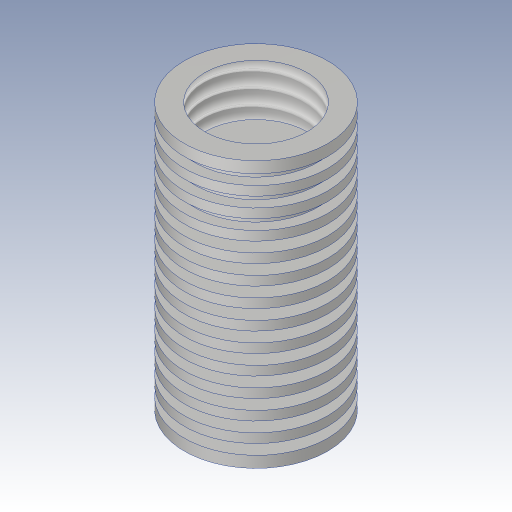
# Autodesk Inventor part: BT003_huenin20_23
Saved by Autodesk Inventor 2023.3 (Build 273359000, 359)
## iProperties
Company: HTBLA Kaindorf
RuleStatus: InUse
Created: 2023-08-12
Part Number: BT003_huenin20_23
Project: Fiberprinter-Hotend
Material: Aluminium 6061
Description: Coldend
Document SubType Name: Modeling
Designer: huenin20
Density: 2.7 g/cm^3
Appearance: Aluminium - flach
Mass: 5.305 g
Surface Area: 40.404 cm^2
Volume: 1.96481 cm^3
AfterDocNew0: iProperties-Editor_aufrufen
Author: nicob
Keywords: 2023
Autodesk Inventor part; units mm, degrees
ref_plane "YZ Plane" through (0, 0, 0) normal (1, 0, 0) x (0, 1, 0)
ref_plane "XZ Plane" through (0, 0, 0) normal (0, 1, 0) x (-1, 0, 0)
ref_plane "XY Plane" through (0, 0, 0) normal (0, 0, 1) x (1, 0, 0)
sketch "Skizze3" plane through (0, 0, 0) normal (1, 0, 0) x (0, 1, 0)
  line L0 (-4, 0) -> (-4, 6)
  line L1 (-4, 6) -> (-1, 6)
  line L2 (-1, 6) -> (-1, 8)
  line L3 (-1, 8) -> (-2.1, 8)
  line L4 (-5, 26) -> (-7, 26)
  line L5 (-7, 26) -> (-7, 0)
  line L6 (-7, 0) -> (-4, 0)
  line L7 (0, 0) -> (0, 30.1888)
  line L8 (-2.1, 8) -> (-2.1, 21)
  line L9 (-2.1, 21) -> (-5, 21)
  line L10 (-5, 21) -> (-5, 26)
  point P0 (-5.5, 0)
  dimension "d4" = 8
  dimension "d5" = 2
  dimension "d7" = 6
  dimension "d8" = 2
  dimension "d9" = 14
  dimension "d10" = 26
  dimension "d11" = 10
  dimension "d12" = 5
  dimension "d13" = 4.2
  constraints: 22 end point, 6 perpendicular, 4 vertical, 1 horizontal alignment, 1 midpoint
  measures "d4" diameter of L0.start L7
  measures "d5" diameter of L2 L7
  measures "d7" distance from line of L0.start L1
  measures "d8" distance between parallel lines of L3 L1
  measures "d9" diameter of L5 L7
  measures "d10" distance from line of point (-5.5, 0) L4
  measures "d11" diameter of L10 L7
  measures "d12" distance of L9.end L4.start
  measures "d13" diameter of L8 L7
revolve "Umdrehung1" add sketch "Skizze3" angle 360 about axis through (0, 0, 0) along (0, 0, 1)
thread "Gewinde1" size "M8x1" class "6H" standard "ISO Metric profile" length 5 offset 1
thread "Gewinde2" size "M10x1.5" class "6H" standard "ISO Metric profile" length 5
sketch "Skizze4" plane through (0, 0, 0) normal (1, 0, 0) x (0, 1, 0)
  line L0 (-7, 0) -> (-7, 26) projected
  line L1 (-7, 19.2) -> (-3.5, 19.2)
  line L2 (-7, 19.2) -> (-3.5, 19.2) construction
  line L3 (-3.5, 19.2) -> (-3.5, 18.2)
  line L4 (-3.5, 18.2) -> (-10, 18.2)
  line L5 (5, 21) -> (-5, 21) projected
  line L6 (-7, 17.3) -> (-3.5, 17.3)
  line L7 (-3.5, 16.3) -> (-10, 16.3)
  line L8 (-3.5, 17.3) -> (-3.5, 16.3)
  line L9 (-7, 15.4) -> (-3.5, 15.4)
  line L10 (-3.5, 14.4) -> (-10, 14.4)
  line L11 (-3.5, 15.4) -> (-3.5, 14.4)
  line L12 (-7, 13.5) -> (-3.5, 13.5)
  line L13 (-3.5, 12.5) -> (-10, 12.5)
  line L14 (-3.5, 13.5) -> (-3.5, 12.5)
  line L15 (-7, 11.6) -> (-3.5, 11.6)
  line L16 (-3.5, 10.6) -> (-10, 10.6)
  line L17 (-3.5, 11.6) -> (-3.5, 10.6)
  line L18 (-7, 9.7) -> (-3.5, 9.7)
  line L19 (-3.5, 8.7) -> (-10, 8.7)
  line L20 (-3.5, 9.7) -> (-3.5, 8.7)
  line L21 (-7, 7.8) -> (-3.5, 7.8)
  line L22 (-3.5, 6.8) -> (-10, 6.8)
  line L23 (-3.5, 7.8) -> (-3.5, 6.8)
  line L24 (-7, 13.5) -> (7, 13.5) construction
  line L25 (7, 0) -> (7, 26) projected
  line L26 (-7, 1.1) -> (-5, 1.1)
  line L27 (-5, 1.1) -> (-5, 2.1)
  line L28 (-5, 2.1) -> (-7, 2.1)
  line L29 (7, 0) -> (-7, 0) projected
  line L30 (-5, 4) -> (-7, 4)
  line L31 (-7, 3) -> (-5, 3)
  line L32 (-5, 3) -> (-5, 4)
  line L33 (-5, 5.9) -> (-7, 5.9)
  line L34 (-7, 4.9) -> (-5, 4.9)
  line L35 (-5, 4.9) -> (-5, 5.9)
  line L36 (-7, 20.1) -> (-6, 20.1)
  line L37 (-6, 20.1) -> (-6, 21.1)
  line L38 (-6, 21.1) -> (-7, 21.1)
  line L39 (-6, 23) -> (-7, 23)
  line L40 (-6, 22) -> (-6, 23)
  line L41 (-7, 22) -> (-6, 22)
  line L42 (-6, 24.9) -> (-7, 24.9)
  line L43 (-6, 23.9) -> (-6, 24.9)
  line L44 (-7, 23.9) -> (-6, 23.9)
  line L45 (0, 0) -> (0, 30.1888) projected
  line L46 (-2.1, 21) -> (-2.1, 8) projected
  line L47 (-5, 26) -> (-5, 21) projected
  line L48 (-4, 6) -> (-4, 0) projected
  point P0 (-7, 4.9)
  point P1 (-7, 6.8)
  point P2 (-7, 8.7)
  point P3 (-7, 11.6)
  point P4 (-7, 10.6)
  point P5 (-7, 12.5)
  point P6 (-7, 14.4)
  point P7 (-7, 18.2)
  point P8 (-7, 16.3)
  point P9 (-7, 22)
  point P10 (-7, 24.9)
  point P11 (-7, 4)
  dimension "d21" = 1
  dimension "d22" = 1.8
  dimension "d25" = 1.9
  dimension "d31" = 1
  dimension "d32" = 1.1
  dimension "d35" = 1.9
  dimension "d41" = 1
  dimension "d42" = 0.9
  dimension "d45" = 1.9
  dimension "d51" = 1
  dimension "d52" = 1.4
  dimension "d53" = 1
  constraints: 82 end point, 40 vertical alignment, 20 parallel, 11 collinear, 7 horizontal, 4 perpendicular, 1 point on line, 6 other
  measures "d21" distance of L1.end L3.end
  measures "d22" distance between parallel lines of L5 L1
  measures "d25" distance of L1.start L6.start
  measures "d31" distance of L26.end L27.end
  measures "d32" distance between parallel lines of L29 L26
  measures "d35" distance of L27.end L30.start
  measures "d41" distance of L36.end L37.end
  measures "d42" distance between parallel lines of L1 L36
  measures "d45" distance of L37.end L39.start
  measures "d51" distance between parallel lines of L47 L37
  measures "d52" distance between parallel lines of L46 L3
  measures "d53" distance between parallel lines of L48 L27
revolve "Umdrehung2" cut sketch "Skizze4" angle 360 about axis through (0, 0, 0) along (0, 0, 1)
